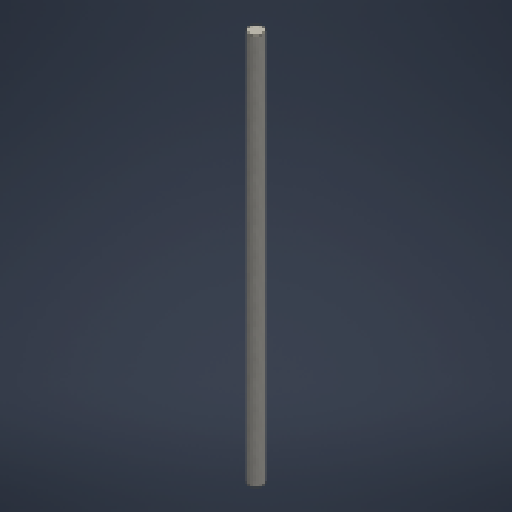
# Autodesk Inventor part: Rod_400x10_V1
Saved by Autodesk Inventor 2024.1 (Build 281209000, 209)
## iProperties
Created: 2022-11-22
Part Number: Rod_400x10_V1
Material: Steel, Cast
Document SubType Name: Modeling
Designer: jaege
Density: 7.85 g/cm^3
Appearance: Steel - Cast
Author: jaege
Autodesk Inventor part; units mm, degrees
ref_plane "YZ Plane" through (0, 0, 0) normal (1, 0, 0) x (0, 1, 0)
ref_plane "XZ Plane" through (0, 0, 0) normal (0, 1, 0) x (-1, 0, 0)
ref_plane "XY Plane" through (0, 0, 0) normal (0, 0, 1) x (1, 0, 0)
sketch "Sketch1" plane through (0, 0, 0) normal (0, 1, 0) x (-1, 0, 0)
  circle A0 centre (0, 0) radius 5
  dimension "d0" = 10
  constraints: 1 centre point, 1 coincident
  measures "d0" diameter of A0
extrude "Extrusion1" add sketch "Sketch1" along normal blind 300
thread "Thread1" size "TR10x2" class "7e" standard "ISO Metric Trapezoidal Threads" full length
body "Solid1"
